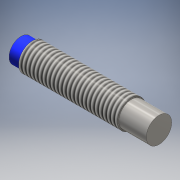
# Autodesk Inventor part: LJ12A3-4-Z Sensor
Saved by Autodesk Inventor 2016 (Build 200138000, 138)
## iProperties
Created: 2017-03-21
Part Number: LJ12A3-4-Z Sensor
Material: Stainless Steel
Document SubType Name: Modeling
Designer: Scott
Density: 8 g/cm^3
Appearance: Semi-Polished
Author: Scott
Autodesk Inventor part; units mm, degrees
ref_plane "YZ Plane" through (0, 0, 0) normal (1, 0, 0) x (0, 1, 0)
ref_plane "XZ Plane" through (0, 0, 0) normal (0, 1, 0) x (-1, 0, 0)
ref_plane "XY Plane" through (0, 0, 0) normal (0, 0, 1) x (1, 0, 0)
sketch "Sketch1" plane through (0, 0, 0) normal (0, 0, 1) x (1, 0, 0)
  line L0 (0, 0) -> (60, 0)
  line L1 (60, 0) -> (60, 5.5)
  line L2 (60, 5.5) -> (48, 5.5)
  line L3 (48, 5.5) -> (48, 6)
  line L4 (48, 6) -> (5, 6)
  line L5 (5, 6) -> (5, 5.2)
  line L6 (5, 5.2) -> (0, 5.2)
  line L7 (0, 5.2) -> (0, 0)
  dimension "d0" = 5.2
  dimension "d1" = 5.5
  dimension "d2" = 6
  dimension "d3" = 5
  dimension "d4" = 48
  dimension "d5" = 60
  constraints: 16 end point, 7 perpendicular, 1 horizontal
  measures "d0" distance of L6.end L0.start
  measures "d1" distance between parallel lines of L0 L2
  measures "d2" distance between parallel lines of L0 L4
  measures "d3" distance of L5.end L6.end
  measures "d4" distance from line of L7 L3.end
  measures "d5" distance of L0.start L0.end
revolve "Revolution1" add sketch "Sketch1" angle 360 about axis through (0, 0, 0) along (1, 0, 0)
thread "Thread1" size "M12x1.75" class "6g" standard "ANSI Metric M Profile" full length
body "Solid1"
